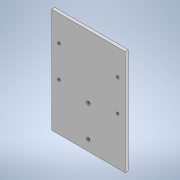
# Autodesk Inventor part: 20220613_カメラ固定
Saved by Autodesk Inventor 2020 (Build 240168000, 168)
## iProperties
Created: 2022-06-13
Part Number: 20220613_カメラ固定
Material: 一般
Document SubType Name: Modeling
Designer: Naggy
Density: 1 g/cm^3
Appearance: 既定
Author: Naggy
Autodesk Inventor part; units mm, degrees
ref_plane "YZ Plane" through (0, 0, 0) normal (1, 0, 0) x (0, 1, 0)
ref_plane "XZ Plane" through (0, 0, 0) normal (0, 1, 0) x (-1, 0, 0)
ref_plane "XY Plane" through (0, 0, 0) normal (0, 0, 1) x (1, 0, 0)
sketch "スケッチ1" plane through (0, 0, 0) normal (0, 0, 1) x (1, 0, 0)
  line L0 (-35, -50) -> (35, -50)
  line L1 (35, -50) -> (35, 50)
  line L2 (35, 50) -> (-35, 50)
  line L3 (-35, 50) -> (-35, -50)
  line L4 (-35, -50) -> (35, 50) construction
  line L5 (35, -50) -> (-35, 50) construction
  point P0 (0, 0)
  dimension "d0" = 70
  dimension "d1" = 100
  constraints: 12 end point, 2 midpoint, 2 parallel, 1 horizontal, 1 perpendicular
  measures "d0" distance between parallel lines of L3 L1
  measures "d1" distance between parallel lines of L0 L2
extrude "押し出し1" add sketch "スケッチ1" along normal blind 3
sketch "スケッチ2" plane through (0, 0, 3) normal (0, 0, 1) x (1, 0, 0)
  line L0 (-35, -50) -> (35, -50) projected
  point P0 (0, 0)
  point P1 (0, -40)
  point P2 (0, -10)
  dimension "d4" = 10
  dimension "d5" = 30
  measures "d4" distance from line of L0 point (0, -40)
  measures "d5" distance of point (0, -10) point (0, -40)
hole "穴1" at (0, -40, 3) at (0, -10, 3) direction (0, 0, -1) diameter 3.2 depth 8.8 tip angle 118
sketch "スケッチ3" plane through (0, 0, 3) normal (0, 0, 1) x (1, 0, 0)
  line L0 (-35, 50) -> (-35, -50) projected
  line L1 (35, -50) -> (35, 50) projected
  point P0 (0, 0)
  point P1 (-28, 25.3325)
  point P2 (28, 25.3325)
  point P3 (-28, -4.6675)
  point P4 (28, -4.6675)
  dimension "d14" = 7
  dimension "d15" = 7
  dimension "d16" = 30
  dimension "d17" = 30
  dimension "d18" = 56
  measures "d14" distance from line of L0 point (-28, 25.332)
  measures "d15" distance from line of point (28, 25.332) L1
  measures "d16" distance of point (-28, -4.668) point (-28, 25.332)
  measures "d17" distance of point (28, -4.668) point (28, 25.332)
  measures "d18" distance of point (28, -4.668) point (-28, -4.668)
hole "穴2" at (-28, 25.3325, 3) at (28, 25.3325, 3) at (-28, -4.6675, 3) at (28, -4.6675, 3) direction (0, 0, -1) diameter 2.459 depth 8.8 tip angle 118 thread size "M3x0.5" class "6H" standard "ISO Metric profile"
